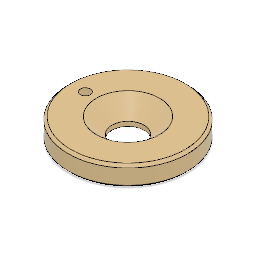
specimen carousel assembly v22 (Autodesk Fusion 360 archive; units mm, degrees)
design "BC vertical rod endcap"
Autodesk Fusion 360 part; units mm, degrees
note: some values were not read from the file. Set by a fixed rule: the direction of a hole.
cylinder "CylinderPrimitive1" add diameter 23.8 height 4 placed x (1, 0, 0) y (0, 0, -1) z (0, 1, 0) at (0, 0, 0)
hole "Hole1" at (0, 4, 0) direction (0, -1, 0) diameter 6.4 end through all countersink diameter 12.6 countersink angle 90
chamfer "Chamfer1" distance 0.5 angle 45 2 edges at (-11.0947, 4, 4.3032) (-11.0947, 0, -4.3032)
sketch "Sketch4" plane through (0, 0, 0) normal (0, 1, 0) x (1, 0, 0)
  circle A0 centre (0, 0) radius 8.5 construction
  point P0 (-8.5, 0)
  dimension "d9" = 17
  constraint coincident A0.centre origin
  constraint coincident A0 P0
  constraint horizontal A0.centre P0
  measures "d9" diameter of A0
hole "Hole2" at (-8.5, 0, 0) direction (0, 1, 0) diameter 2 end through all

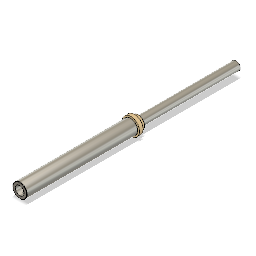
design "BC vertical rod"
Autodesk Fusion 360 part; units mm, degrees
sketch "Sketch1" plane through (0, 0, 0) normal (0, 1, 0) x (1, 0, 0)
  line L0 (0, 0) -> (6, 0)
  line L1 (6, 0) -> (6, -145)
  line L2 (6, -145) -> (10, -145)
  line L3 (10, -145) -> (10, -297.5)
  line L4 (10, -297.5) -> (0, -297.5)
  line L5 (0, -297.5) -> (0, 0)
  line L6 (10, -145) -> (12, -145)
  line L7 (12, -145) -> (12, -140)
  line L8 (12, -140) -> (9, -140)
  line L9 (9, -140) -> (9, -135)
  line L10 (9, -135) -> (6, -135)
  dimension "d1" = 10
  dimension "d2" = 6
  dimension "d3" = 145
  dimension "d4" = 152.5
  dimension "d12" = 5
  dimension "d13" = 9
  dimension "d14" = 12
  dimension "d15" = 5
  constraint coincident L0.start L5.end
  constraint horizontal L0
  constraint perpendicular L0 L1
  constraint perpendicular L1 L2
  constraint perpendicular L2 L3
  constraint perpendicular L3 L4
  constraint vertical L5
  constraint perpendicular L3 L6
  constraint perpendicular L6 L7
  constraint perpendicular L3 L8
  constraint perpendicular L6 L9
  constraint coincident L1 L10.end
  constraint perpendicular L1 L10
  measures "d1" distance of L3 L5
  measures "d2" distance of L1 L5
  measures "d3" distance of L0 L2
  measures "d4" distance of L2 L4
  measures "d12" distance of L6 L8
  measures "d13" distance of L5 L9
  measures "d14" distance of L5 L7
  measures "d15" distance of L8 L10
revolve "Revolve1" add sketch "Sketch1" angle 360 about axis through (0, 0, 297.5) along (0, 0, -1) contours L0 L1 L2 L3 L4 L5 makes body 1
hole "Hole1" at (0, 0, 297.5) direction (0, 0, -1) diameter 12 depth 35 tip angle 118 bodies 1
hole "Hole2" at (0, 0, 297.5) direction (0, 0, -1) diameter 5.035 depth 50 tip angle 118 bodies 1
thread "Thread1" "ISO Metric profile 6.0 M6x1 6H"
hole "Hole3" at (0, 0, 0) direction (0, 0, 1) diameter 5.035 depth 25 tip angle 118 bodies 1
thread "Thread2" "ISO Metric profile 6.0 M6x1 6H"
chamfer "Chamfer1" distance 0.5 angle 45 3 edges at (-5.594, -2.1697, 0) (-9.3233, -3.6162, 145) (-9.3233, -3.6162, 297.5) on bodies 1
revolve "Revolve2" add sketch "Sketch1" angle 360 about axis through (0, 0, 1.75) along (0, 0, 1) separate body contours L1 L2 L6 L7 L8 L9 L10 makes body 2
sketch "Sketch2" plane through (0, 0, 0) normal (0, 1, 0) x (1, 0, 0)
  line L0 (2.5175, -247.5) -> (-2.5175, -247.5)
  line L1 (2.5175, -260.4075) -> (-2.5175, -260.4075)
  line L2 (9.5, -297.5) -> (-9.5, -297.5)
  point P0 (0, -247.5)
  point P1 (0, -260.4075)
  point P2 (0, -25)
  point P3 (0, -280)
  point P4 (0, -290)
  dimension "d24" = 10
  dimension "d25" = 7.5
  constraint midpoint P0 L0
  constraint midpoint P1 L1
  constraint vertical P3 P4
  constraint vertical origin P3
  measures "d24" distance of P3 P4
  measures "d25" distance of P4 L2
hole "Hole4" at (0, 0, 25) at (0, 0, 247.5) at (0, 0, 260.4075) direction (0, -1, 0) diameter 3 end through all bodies 1
copy_body "Body->Comp1" bodies 1 removing the originals makes body 3 in component "vertical rod"
copy_body "Body->Comp2" bodies 2 removing the originals makes body 4 in component "peek insulator"
hole "Hole1'" at (0, 0, 280) at (0, 0, 290) direction (0, -1, 0) diameter 4.234 end through all bodies 3 in component "vertical rod"
thread "Thread1'" "ISO Metric profile 5.0 M5x0.8 6H" in component "vertical rod"
component "vertical rod" placed x (1, 0, 0) y (0, 1, 0) z (0, 0, 1) at (0, 0, 0)
component "peek insulator" placed x (1, 0, 0) y (0, 1, 0) z (0, 0, 1) at (0, 0, 0)
equation "d4 = 117.5 mm + 35 mm"
named bodies: "vertical rod", "peek insulator"
